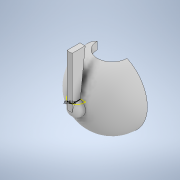
# Autodesk Inventor part: Head back
Saved by Autodesk Inventor 2020 (Build 240168000, 168)
## iProperties
Created: 2022-05-04
Part Number: Head back
Material: Generic
Document SubType Name: Modeling
Designer: Administrator
Density: 1 g/cm^3
Appearance: Default
Author: Administrator
Autodesk Inventor part; units mm, degrees
sketch "Sketch1" plane through (0, 0, 0) normal (0, 0, 1) x (1, 0, 0)
  arc A0 (0, -8.6995) -> (0, 8.6995) centre (0, 0) ccw
  line L0 (0, 8.6995) -> (0, -8.6995)
  dimension "d0" = 17.399
  constraints: 2 end point, 2 point on circle, 1 centre point, 1 coincident, 1 vertical
  measures "d0" diameter of A0
revolve "Revolution1" add sketch "Sketch1" angle 180 about axis through (0, 8.6995, 0) along (0, -1, 0)
shell "Shell1" thickness 1.651 removed faces 2 at (4.2263, 0.0174, 0) at (-4.2263, 0.0174, 0)
ref_plane "Work Plane1" through (0, 8.6995, 0) normal (0, 1, 0) x (-1, 0, 0)
sketch "Sketch2" plane through (0, 8.6995, 0) normal (0, 1, 0) x (-1, 0, 0)
  circle A0 centre (0, 0) radius 3.683
  dimension "d4" = 7.366
  constraints: 1 centre point, 1 coincident
  measures "d4" diameter of A0
extrude "Extrusion1" cut sketch "Sketch2" against normal blind 5.08
sketch "Sketch3" plane through (0, 0, 0) normal (0, 0, -1) x (-1, 0, 0)
  circle A0 centre (-5.969, 0) radius 1.0795
  arc A1 (-3.683, 6.0097) -> (3.683, 6.0097) centre (0, 0) ccw projected
  circle A2 centre (-5.969, 0) radius 1.7145
  circle A3 centre (5.969, 0) radius 1.0795
  circle A4 centre (5.969, 0) radius 1.7145
  point P0 (6.8999, 1.4398)
  point P1 (6.8999, -1.4398)
  point P2 (7.0485, 0)
  point P3 (-6.8999, 1.4398)
  point P4 (-7.0485, 0)
  point P5 (-6.8999, -1.4398)
  dimension "d7" = 2.159
  dimension "d8" = 0.635
  dimension "d9" = 2.159
  dimension "d10" = 0.635
  constraints: 4 centre point, 2 tangent
  measures "d7" diameter of A0
  measures "d8" radial gap between concentric circles of A0 A2
  measures "d9" diameter of A3
  measures "d10" radial gap between concentric circles of A3 A4
extrude "Extrusion2" add sketch "Sketch3" against normal up to next contours A1 A2 | A4 A1 picked at (-6.1111, -1.368) picked at (6.7446, 1.1376)
ref_plane "Work Plane2" through (0, 0, 2.032) normal (0, 0, -1) x (-1, 0, 0)
sketch "Sketch6" plane through (0, 0, 2.032) normal (0, 0, -1) x (-1, 0, 0)
  circle A0 centre (0, 0) radius 2.54
  circle A1 centre (0, 0) radius 0.9525
  dimension "d14" = 5.08
  dimension "d15" = 1.905
  constraints: 2 centre point, 2 coincident
  measures "d14" diameter of A0
  measures "d15" diameter of A1
extrude "Extrusion3" add sketch "Sketch6" against normal blind 6.096
ref_plane "Work Plane3" through (0, 0, 8.6995) normal (0, 0, -1) x (-1, 0, 0)
sketch "Sketch7" plane through (0, 0, 8.6995) normal (0, 0, -1) x (-1, 0, 0)
  circle A0 centre (0, 0) radius 0.9525 projected
  arc A1 (1.905, 0) -> (-1.905, 0) centre (0, 0) ccw
  line L0 (1.905, 0) -> (-1.905, 0)
  dimension "d19" = 3.81
  constraints: 2 end point, 2 point on circle, 1 centre point, 1 coincident, 1 horizontal
  measures "d19" diameter of A1
revolve "Revolution2" add sketch "Sketch7" angle 360 about axis through (-1.905, 0, 8.6995) along (1, 0, 0) picked at (0.2377, 0.2105) contours L0 A0 | A0 L0 A1
sketch "Sketch8" plane through (0, 0, 2.032) normal (0, 0, -1) x (-1, 0, 0)
  circle A0 centre (0, 0) radius 0.9525 projected
  circle A1 centre (0, 0) radius 0.9525
  constraints: 1 centre point, 1 coincident
extrude "Extrusion4" cut sketch "Sketch8" against normal blind 6.096
ref_plane "Work Plane4" through (0, 1.905, 0) normal (0, 1, 0) x (-1, 0, 0)
sketch "Sketch9" plane through (0, 1.905, 0) normal (0, 1, 0) x (-1, 0, 0)
  arc A0 (1.8935, 8.4909) -> (-1.8935, 8.4909) centre (0, 8.6995) ccw projected
  line L0 (0, 10.6045) -> (0.635, 10.6045)
  line L1 (0, 10.6045) -> (-0.635, 10.6045)
  line L2 (-0.635, 10.6045) -> (-0.635, 8.4909)
  line L3 (-1.8935, 8.4909) -> (1.8935, 8.4909) projected
  line L4 (0.635, 10.6045) -> (0.635, 8.4909)
  point P0 (0, 0)
  point P1 (0.635, 10.4956)
  point P2 (-0.635, 10.4956)
  dimension "d24" = 0.635
  dimension "d25" = 0.635
  constraints: 8 end point, 2 point on line, 1 collinear, 1 horizontal, 1 parallel, 1 point on circle, 1 tangent, 1 vertical
  measures "d24" distance of L0.start L0.end
  measures "d25" distance of L0.start L1.end
extrude "Extrusion5" add sketch "Sketch9" against normal blind 1.905 contours L4 L3 L2 A0
ref_plane "Work Plane5" through (0, 12.7, 0) normal (0, 1, 0) x (-1, 0, 0)
sketch "Sketch10" plane through (0, 12.7, 0) normal (0, 1, 0) x (-1, 0, 0)
  line L0 (0.635, 8.4909) -> (0.635, 10.4956) projected
  line L1 (-0.635, 10.4956) -> (-0.635, 8.4909) projected
  line L2 (0.635, 10.4956) -> (-0.635, 10.4956)
  line L3 (-0.635, 10.4956) -> (-0.635, 7.3206)
  line L4 (-0.635, 7.3206) -> (0.635, 7.3206)
  line L5 (0.635, 7.3206) -> (0.635, 10.4956)
  arc A0 (0.635, 10.4956) -> (-0.635, 10.4956) centre (0, 8.6995) ccw
  point P0 (0, 0)
  dimension "d29" = 3.175
  constraints: 8 end point, 2 perpendicular, 2 point on circle, 1 centre point, 1 collinear, 1 horizontal
  measures "d29" distance of L1.start L3.end
loft "Loft1" add profiles "Sketch10" section 1 edges at (0, 1.905, 10.6045) (0.635, 1.905, 9.4932) (0, 1.905, 8.4909) (-0.635, 1.905, 9.4932)
body "Solid1"
